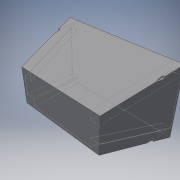
# Autodesk Inventor part: Front Cover
Saved by Autodesk Inventor 2019 (Build 230136000, 136)
## iProperties
Created: 2018-10-04
Part Number: Front Cover
Material: Generic
Document SubType Name: Modeling
Designer: Adhik
Density: 1 g/cm^3
Appearance: Default
Mass: 1256.97 g
Surface Area: 4470.16 cm^2
Volume: 1256.97 cm^3
Author: Adhik
Autodesk Inventor part; units mm, degrees
ref_plane "YZ Plane" through (0, 0, 0) normal (1, 0, 0) x (0, 1, 0)
ref_plane "XZ Plane" through (0, 0, 0) normal (0, 1, 0) x (-1, 0, 0)
sketch "Sketch1" plane through (0, 0, 0) normal (0, 0, 1) x (1, 0, 0)
  line L0 (-251.1425, 0) -> (251.1425, 0) construction
  line L1 (0, -146.685) -> (0, 146.685) construction
  line L2 (-179.3875, 104.775) -> (179.3875, 104.775)
  line L3 (179.3875, 104.775) -> (179.3875, -104.775)
  line L4 (179.3875, -104.775) -> (-179.3875, -104.775)
  line L5 (-179.3875, -104.775) -> (-179.3875, 104.775)
  point P0 (0, 0)
  point P1 (0, 104.775)
  point P2 (-179.3875, 0)
  dimension "d0" = 358.775
  dimension "d1" = 209.55
  constraints: 8 end point, 2 midpoint, 2 parallel, 2 point on line, 1 horizontal, 1 perpendicular
  measures "d0" distance of L2.start L2.end
  measures "d1" distance of L4.end L2.start
ref_plane "Work Plane1" through (0, 0, 203.2) normal (0, 0, 1) x (1, 0, 0)
sketch "Sketch2" plane through (0, 0, 203.2) normal (0, 0, 1) x (1, 0, 0)
  line L0 (0, -146.685) -> (0, 146.685) construction
  line L1 (-253.365, 0) -> (253.365, 0) construction
  line L2 (-128.5875, 53.975) -> (128.5875, 53.975)
  line L3 (128.5875, 53.975) -> (128.5875, -53.975)
  line L4 (128.5875, -53.975) -> (-128.5875, -53.975)
  line L5 (-128.5875, -53.975) -> (-128.5875, 53.975)
  line L6 (-179.3875, 104.775) -> (179.3875, 104.775) construction
  line L7 (-179.3875, -104.775) -> (-179.3875, 104.775) construction
  point P0 (0, 0)
  point P1 (0, 53.975)
  point P2 (-128.5875, 0)
  dimension "d3" = 50.8
  dimension "d4" = 50.8
  constraints: 8 end point, 2 midpoint, 2 parallel, 2 point on line, 1 horizontal, 1 perpendicular
  measures "d3" distance between parallel lines of L6 L2
  measures "d4" distance between parallel lines of L7 L5
loft "Loft1" add profiles "Sketch1", "Sketch2"
sketch "Sketch3" plane through (179.3875, 104.775, 0) normal (0, 0, -1) x (-1, 0, 0)
  line L0 (179.3875, -251.46) -> (179.3875, 41.91) construction
  line L1 (430.53, -104.775) -> (-71.755, -104.775) construction
  line L2 (3.175, -3.175) -> (28.575, -3.175) construction
  line L3 (355.6, -3.175) -> (355.6, -28.575) construction
  line L4 (355.6, -206.375) -> (330.2, -206.375) construction
  line L5 (3.175, -206.375) -> (3.175, -180.975) construction
  line L6 (28.575, -3.175) -> (28.575, -28.575)
  line L7 (28.575, -28.575) -> (3.175, -28.575)
  line L8 (3.175, -180.975) -> (28.575, -180.975)
  line L9 (28.575, -180.975) -> (28.575, -206.375)
  line L10 (330.2, -3.175) -> (330.2, -28.575)
  line L11 (330.2, -28.575) -> (355.6, -28.575)
  line L12 (330.2, -206.375) -> (330.2, -180.975)
  line L13 (330.2, -180.975) -> (355.6, -180.975)
  line L14 (3.175, -28.575) -> (3.175, -3.175) construction
  line L15 (28.575, -3.175) -> (330.2, -3.175)
  line L16 (330.2, -3.175) -> (355.6, -3.175) construction
  line L17 (355.6, -28.575) -> (355.6, -180.975)
  line L18 (355.6, -180.975) -> (355.6, -206.375) construction
  line L19 (330.2, -206.375) -> (28.575, -206.375)
  line L20 (28.575, -206.375) -> (3.175, -206.375) construction
  line L21 (3.175, -180.975) -> (3.175, -28.575)
  line L22 (0, 0) -> (0, -209.55) construction
  line L23 (358.775, 0) -> (0, 0) construction
  point P0 (179.3875, -104.775)
  point P1 (179.3875, -3.175)
  point P2 (3.175, -104.775)
  dimension "d9" = 3.175
  dimension "d10" = 3.175
  dimension "d11" = 25.4
  constraints: 40 end point, 19 parallel, 18 perpendicular, 11 point on line, 3 equal length, 3 horizontal, 2 midpoint, 1 collinear, 1 vertical
  measures "d9" distance between parallel lines of L22 L14
  measures "d10" distance between parallel lines of L23 L2
  measures "d11" distance of L2.end L6.end
ref_plane "Work Plane2" through (0, 0, 200.025) normal (0, 0, 1) x (1, 0, 0)
sketch "Sketch5" plane through (0, 0, 200.025) normal (0, 0, 1) x (1, 0, 0)
  line L0 (150.8125, 101.6) -> (150.8125, 76.2) projected
  line L1 (150.8125, 76.2) -> (176.2125, 76.2) projected
  line L2 (176.2125, -76.2) -> (176.2125, 76.2) projected
  line L3 (176.2125, -76.2) -> (150.8125, -76.2) projected
  line L4 (150.8125, -76.2) -> (150.8125, -101.6) projected
  line L5 (-150.8125, -101.6) -> (150.8125, -101.6) projected
  line L6 (-150.8125, -101.6) -> (-150.8125, -76.2) projected
  line L7 (-150.8125, -76.2) -> (-176.2125, -76.2) projected
  line L8 (-176.2125, 76.2) -> (-176.2125, -76.2) projected
  line L9 (-150.8125, 76.2) -> (-176.2125, 76.2) projected
  line L10 (-150.8125, 101.6) -> (-150.8125, 76.2) projected
  line L11 (150.8125, 101.6) -> (-150.8125, 101.6) projected
  line L12 (-100.0125, 50.8) -> (-100.0125, 25.4)
  line L13 (-100.0125, 25.4) -> (-125.4125, 25.4)
  line L14 (-125.4125, 25.4) -> (-125.4125, -25.4)
  line L15 (-125.4125, -25.4) -> (-100.0125, -25.4)
  line L16 (-100.0125, -25.4) -> (-100.0125, -50.8)
  line L17 (-100.0125, -50.8) -> (100.0125, -50.8)
  line L18 (100.0125, -50.8) -> (100.0125, -25.4)
  line L19 (100.0125, -25.4) -> (125.4125, -25.4)
  line L20 (125.4125, -25.4) -> (125.4125, 25.4)
  line L21 (125.4125, 25.4) -> (100.0125, 25.4)
  line L22 (100.0125, 25.4) -> (100.0125, 50.8)
  line L23 (100.0125, 50.8) -> (-100.0125, 50.8)
  line L24 (-128.5875, 53.975) -> (128.5875, 53.975) projected
  point P0 (0, 0)
  dimension "d15" = 3.175
  constraints: 24 end point, 11 other
  measures "d15" distance between parallel lines of L24 L23
loft "Loft2" cut profiles "Sketch3", "Sketch5" contours all / L23 L22 L21 L20 L19 L18 L17 L16 L15 L14 L13 L12
sketch "Sketch6" plane through (179.3875, 104.775, 0) normal (0, 0, -1) x (-1, 0, 0)
  line L0 (430.53, -104.775) -> (-71.755, -104.775) construction
  line L1 (179.3875, -251.46) -> (179.3875, 41.91) construction
  line L2 (15.875, -15.875) -> (342.9, -15.875) construction
  line L3 (342.9, -15.875) -> (342.9, -193.675) construction
  line L4 (342.9, -193.675) -> (15.875, -193.675) construction
  line L5 (15.875, -193.675) -> (15.875, -15.875) construction
  line L6 (3.175, -28.575) -> (28.575, -28.575) construction
  line L7 (28.575, -28.575) -> (28.575, -3.175) construction
  circle A0 centre (15.875, -15.875) radius 3.175
  circle A1 centre (342.9, -15.875) radius 3.175
  circle A2 centre (342.9, -193.675) radius 3.175
  circle A3 centre (15.875, -193.675) radius 3.175
  point P0 (179.3875, -104.775)
  point P1 (179.3875, -15.875)
  point P2 (15.875, -104.775)
  dimension "d20" = 12.7
  dimension "d21" = 12.7
  dimension "d22" = 6.35
  constraints: 8 end point, 4 centre point, 4 coincident, 3 equal radius, 2 midpoint, 2 parallel, 2 point on line, 1 horizontal, 1 perpendicular
  measures "d20" distance between parallel lines of L6 L2
  measures "d21" distance between parallel lines of L7 L5
  measures "d22" diameter of A0
extrude "Extrusion1" cut sketch "Sketch6" against normal through all
equation "\"d21\" = d20"
body "Solid1"
